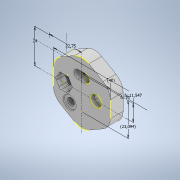
# Autodesk Inventor part: Bottom
Saved by Autodesk Inventor 2022 (Build 260153000, 153)
## iProperties
Created: 2021-02-26
Part Number: Bottom
Material: Generic
Document SubType Name: Modeling
Designer: Viktor
Density: 1 g/cm^3
Appearance: Default
Author: Viktor
Autodesk Inventor part; units mm, degrees
ref_plane "YZ Plane" through (0, 0, 0) normal (1, 0, 0) x (0, 1, 0)
ref_plane "XZ Plane" through (0, 0, 0) normal (0, 1, 0) x (-1, 0, 0)
ref_plane "XY Plane" through (0, 0, 0) normal (0, 0, 1) x (1, 0, 0)
sketch "Sketch1" plane through (0, 0, 0) normal (0, 0, 1) x (1, 0, 0)
  circle A0 centre (0, 0) radius 7.5
  line L0 (-5.7735, 0) -> (-2.8868, 5)
  line L1 (-2.8868, 5) -> (2.8868, 5)
  line L2 (2.8868, 5) -> (5.7735, 0)
  line L3 (5.7735, 0) -> (2.8868, -5)
  line L4 (2.8868, -5) -> (-2.8868, -5)
  line L5 (-2.8868, -5) -> (-5.7735, 0)
  dimension "d0" = 15
  dimension "d1" = 10
  constraints: 12 end point, 2 coincident, 1 centre point, 13 other
  measures "d0" diameter of A0
  measures "d1" distance between parallel lines of L3 L0
extrude "Extrusion1" add sketch "Sketch1" along normal blind 9 contours A0 | L0 L1 L2 L3 L4 L5
sketch "Sketch4" plane through (0, 0, 9) normal (0, 0, 1) x (1, 0, 0)
  circle A0 centre (0, 0) radius 3
  dimension "d15" = 6
  constraints: 1 centre point, 1 coincident
  measures "d15" diameter of A0
extrude "Extrusion4" cut sketch "Sketch4" against normal through all
sketch "Sketch5" plane through (0, 0, 9) normal (0, 0, 1) x (1, 0, 0)
  line L0 (-2.9156, -5.05) -> (-5.8312, 0)
  line L1 (-5.8312, 0) -> (-2.9156, 5.05)
  line L2 (-2.9156, 5.05) -> (2.9156, 5.05)
  line L3 (2.9156, 5.05) -> (5.8312, 0)
  line L4 (5.8312, 0) -> (2.9156, -5.05)
  line L5 (2.9156, -5.05) -> (-2.9156, -5.05)
  point P0 (0, 0)
  point P1 (0, 0)
  dimension "d18" = 10.1
  constraints: 12 end point, 1 coincident, 1 horizontal, 13 other
  measures "d18" distance between parallel lines of L5 L2
extrude "Extrusion5" cut sketch "Sketch5" against normal blind 6
sketch "Sketch6" plane through (0, 0, 9) normal (0, 0, 1) x (1, 0, 0)
  point P0 (0, 0)
fillet "Fillet1" radius 2.1 6 edges at (5.8312, 0, 6) (2.9156, 5.05, 6) (-2.9156, 5.05, 6) (-5.8312, 0, 6) (-2.9156, -5.05, 6) (2.9156, -5.05, 6)
sketch "Sketch7" plane through (0, 0, 9) normal (0, 0, 1) x (1, 0, 0)
  arc A0 (-3.5218, -4) -> (-1.7032, -5.05) centre (-1.7032, -2.95) ccw projected
  arc A1 (-5.225, 1.05) -> (-5.225, -1.05) centre (-3.4064, 0) ccw projected
  arc A2 (-1.7032, 5.05) -> (-3.5218, 4) centre (-1.7032, 2.95) ccw projected
  arc A3 (3.5218, 4) -> (1.7032, 5.05) centre (1.7032, 2.95) ccw projected
  arc A4 (5.225, -1.05) -> (5.225, 1.05) centre (3.4064, 0) ccw projected
  arc A5 (1.7032, -5.05) -> (3.5218, -4) centre (1.7032, -2.95) ccw projected
  line L0 (-45.8, 0) -> (57.8, 0) projected
  circle A6 centre (-4.6441, 0) radius 1.2
  point P0 (0, 0)
  dimension "d22" = 2.4
  constraints: 1 point on line, 3 other
extrude "Extrusion6" cut sketch "Sketch7" against normal up to surface (6 mm away)
pattern_circular "Circular Pattern1" count 6 over 360 about axis through (0, 0, 9) along (0, 0, -1) of "Extrusion6"
sketch "Sketch9" plane through (0, 0, 0) normal (0, 0, 1) x (1, 0, 0)
  line L0 (-10.5, 0) -> (10.5, 0) projected
  circle A0 centre (12.5, 0) radius 20 construction
  circle A1 centre (0, 0) radius 7.5 projected
  line L1 (-7.5, -11.547) -> (-7.5, 11.547)
  line L2 (-7.5, 11.547) -> (12.5, 23.094)
  line L3 (12.5, 23.094) -> (32.5, 11.547)
  line L4 (32.5, 11.547) -> (32.5, -11.547)
  line L5 (32.5, -11.547) -> (12.5, -23.094)
  line L6 (12.5, -23.094) -> (-7.5, -11.547)
  point P0 (-7.5, 0)
  point P1 (-7.5, 0)
  dimension "d28" = 40
  constraints: 12 end point, 2 tangent, 1 centre point, 1 coincident, 1 point on line, 1 vertical, 13 other
  measures "d28" diameter of A0
extrude "Extrusion7" add sketch "Sketch9" along normal up to surface (9 mm away)
sketch "Sketch10" plane through (10, 0, 9) normal (0, 0, 1) x (1, 0, 0)
  circle A0 centre (-6, -10) radius 2 construction
  point P0 (-10, 0)
  dimension "d31" = 4
  dimension "d32" = 4
  dimension "d33" = 10
  constraints: 1 centre point
  measures "d31" diameter of A0
  measures "d32" horizontal distance of point (-10, 0) A0.centre
  measures "d33" vertical distance of point (-10, 0) A0.centre
fillet "Fillet2" radius 10 6 edges at (-7.5, -11.547, 4.5) (12.5, -23.094, 4.5) (32.5, -11.547, 4.5) (-7.5, 11.547, 4.5) (12.5, 23.094, 4.5) (32.5, 11.547, 4.5)
hole "Hole1" at (4, -10, 9) direction (0, 0, -1) diameter 5 end through all counterbore diameter 9 counterbore depth 0.8
sketch "Sketch13" plane through (0, 0, 0) normal (0, 0, -1) x (-1, 0, 0)
  circle A0 centre (-4, -10) radius 2.5 projected
  line L0 (-8.05, -7.6617) -> (-4, -5.3235)
  line L1 (-4, -5.3235) -> (0.05, -7.6617)
  line L2 (0.05, -7.6617) -> (0.05, -12.3383)
  line L3 (0.05, -12.3383) -> (-4, -14.6765)
  line L4 (-4, -14.6765) -> (-8.05, -12.3383)
  line L5 (-8.05, -12.3383) -> (-8.05, -7.6617)
  line L6 (2.5, -14.4338) -> (-7.5, -20.2073) projected
  point P0 (0, 0)
  point P1 (-6.025, -13.5074)
  dimension "d44" = 8.1
  constraints: 12 end point, 1 coincident, 1 midpoint, 1 parallel, 13 other
  measures "d44" distance between parallel lines of L5 L2
extrude "Extrusion9" cut sketch "Sketch13" against normal blind 5.2
fillet "Fillet3" radius 2.1 6 edges at (4, -14.6765, 2.6) (-0.05, -12.3383, 2.6) (-0.05, -7.6617, 2.6) (4, -5.3235, 2.6) (8.05, -7.6617, 2.6) (8.05, -12.3383, 2.6)
sketch "Sketch15" plane through (0, 0, 0) normal (0, 0, -1) x (-1, 0, 0)
  arc A0 (-5.05, -14.0703) -> (-2.95, -14.0703) centre (-4, -12.2517) ccw projected
  line L0 (-4, -12.2517) -> (-4, -11.6129) construction
  circle A1 centre (-4, -13.3921) radius 1.25
  point P0 (0, 0)
  dimension "d48" = 2.5
  constraints: 2 end point, 1 point on line, 1 vertical, 3 other
extrude "Extrusion10" cut sketch "Sketch15" against normal up to surface (5.2 mm away)
pattern_circular "Circular Pattern2" count 6 over 360 about axis through (4, -10, -50.4819) along (0, 0, 1) of "Extrusion10"
sketch "Sketch16" plane through (0, 0, 9) normal (0, 0, 1) x (1, 0, 0)
  circle A0 centre (22.5, 0) radius 4
  line L0 (32.5, 5.7735) -> (32.5, -5.7735) projected
  point P0 (0, 0)
  dimension "d54" = 8
  dimension "d68" = 10
  constraints: 1 centre point
  measures "d54" diameter of A0
  measures "d68" distance from line of L0 A0.centre
extrude "Extrusion11" cut sketch "Sketch16" against normal through all
sketch "Sketch17" plane through (0, 0, 0) normal (0, 0, -1) x (-1, 0, 0)
  circle A0 centre (-22.5, 0) radius 4 projected
  line L0 (-29.05, -3.7816) -> (-29.05, 3.7816)
  line L1 (-29.05, 3.7816) -> (-22.5, 7.5633)
  line L2 (-22.5, 7.5633) -> (-15.95, 3.7816)
  line L3 (-15.95, 3.7816) -> (-15.95, -3.7816)
  line L4 (-15.95, -3.7816) -> (-22.5, -7.5633)
  line L5 (-22.5, -7.5633) -> (-29.05, -3.7816)
  line L6 (-32.5, -5.7735) -> (-32.5, 5.7735) projected
  point P0 (0, 0)
  dimension "d58" = 13.1
  constraints: 12 end point, 1 coincident, 1 parallel, 13 other
  measures "d58" distance between parallel lines of L0 L3
extrude "Extrusion12" cut sketch "Sketch17" against normal blind 5.5
fillet "Fillet4" radius 2.1 6 edges at (22.5, -7.5633, 2.75) (15.95, -3.7816, 2.75) (15.95, 3.7816, 2.75) (22.5, 7.5633, 2.75) (29.05, 3.7816, 2.75) (29.05, -3.7816, 2.75)
sketch "Sketch19" plane through (0, 0, 0) normal (0, 0, -1) x (-1, 0, 0)
  arc A0 (-23.55, -6.9571) -> (-21.45, -6.9571) centre (-22.5, -5.1384) ccw projected
  line L0 (-22.5, -5.1384) -> (-22.5, -8.2461) construction
  circle A1 centre (-22.5, -6.3761) radius 1.2
  arc A2 (-23.55, -6.9571) -> (-21.45, -6.9571) centre (-22.5, -5.1384) ccw projected
  line L1 (-21.45, -6.9571) -> (-22.5, -7.5633) construction
  line L2 (-23.55, -6.9571) -> (-22.5, -7.5633) construction
  line L3 (-23.55, -6.9571) -> (-28, -4.3879) projected
  point P0 (0, 0)
  dimension "d62" = 2.4
  constraints: 6 end point, 3 point on circle, 2 point on line, 2 tangent, 1 centre point, 1 collinear, 1 vertical
  measures "d62" diameter of A1
extrude "Extrusion13" cut sketch "Sketch19" against normal up to surface (5.5 mm away)
pattern_circular "Circular Pattern3" count 6 over 360 about axis through (22.5, 0, 9) along (0, 0, -1) of "Extrusion13"
sketch "Sketch20" plane through (0, 0, 5.5) normal (0, 0, -1) x (-1, 0, 0)
  circle A0 centre (-22.5, 0) radius 4 projected
  circle A1 centre (-22.5, 0) radius 5.9
  point P0 (0, 0)
  dimension "d69" = 11.8
  constraints: 1 centre point, 1 coincident
  measures "d69" diameter of A1
extrude "Extrusion14" cut sketch "Sketch20" against normal blind 0.65
sketch "Sketch21" plane through (0, 0, 9) normal (0, 0, 1) x (1, 0, 0)
  point P0 (0, 0)
sketch "Sketch22" plane through (0, 0, 9) normal (0, 0, 1) x (1, 0, 0)
  line L0 (54.5318, 10) -> (-19.1234, 10) construction
  arc A0 (32.5, 5.7735) -> (27.5, 14.4338) centre (22.5, 5.7735) ccw projected
  line L1 (-7.5, -5.7735) -> (-7.5, 5.7735) projected
  line L2 (15, 10) -> (10, 10) construction
  line L3 (15, 13) -> (10, 13)
  line L4 (10, 7) -> (15, 7)
  arc A1 (15, 7) -> (15, 13) centre (15, 10) ccw
  arc A2 (10, 13) -> (10, 7) centre (10, 10) ccw
  line L5 (12.5, 32) -> (12.5, -41) construction
  point P0 (0, 0)
  point P1 (12.5, 10)
  dimension "d72" = 40
  dimension "d74" = 6
  dimension "d75" = 5
  dimension "d76" = 10
  dimension "d79" = 20
  constraints: 12 end point, 4 point on circle, 4 tangent, 3 point on line, 2 centre point, 1 horizontal, 1 midpoint, 1 parallel, 1 vertical
  measures "d74" distance between parallel lines of L3 L4
  measures "d75" distance of L4.start L4.end
  measures "d76" vertical distance of point (0, 0) point (12.5, 10)
  measures "d79" distance between parallel lines of L1 L5
extrude "Extrusion15" cut sketch "Sketch22" against normal blind 10
sketch "Sketch23" plane through (0, 0, 9) normal (0, 0, 1) x (1, 0, 0)
  arc A0 (15, 7) -> (15, 13) centre (15, 10) ccw projected
  circle A1 centre (22.5, 0) radius 4 projected
  point P0 (0, 0)
sketch "Sketch24" plane through (0, 0, 0) normal (0, 0, -1) x (-1, 0, 0)
  arc A0 (7.5, 5.7735) -> (2.5, 14.4338) centre (-2.5, 5.7735) ccw projected
  line L0 (7.5, 5.7735) -> (7.5, 22) construction
  line L1 (-10, 7) -> (31, 7) construction
  point P0 (0, 0)
  point P1 (7.5, 7)
  constraints: 4 end point, 2 point on line, 1 coincident, 1 horizontal, 1 tangent, 1 vertical
sketch "Sketch25" plane through (0, 0, 9) normal (0, 0, 1) x (1, 0, 0)
  arc A0 (-2.5, 14.4338) -> (-7.5, 5.7735) centre (2.5, 5.7735) ccw projected
  point P0 (0, 0)
  point P1 (-7.5, 7)
sketch "Sketch26" plane through (0, 0, 0) normal (0, 0, -1) x (-1, 0, 0)
  circle A0 centre (-4, -10) radius 2.5 projected
  circle A1 centre (-22.5, 0) radius 4 projected
  circle A2 centre (0, 0) radius 3 projected
sketch "Sketch27" plane through (0, 0, 0) normal (0, 0, -1) x (-1, 0, 0)
  line L0 (-17, -4.3879) -> (-21.45, -6.9571) projected
  arc A0 (-23.55, -6.9571) -> (-21.45, -6.9571) centre (-22.5, -6.3761) ccw projected
  line L1 (-23.55, -6.9571) -> (-28, -4.3879) projected
  arc A1 (-29.05, -2.5692) -> (-28, -4.3879) centre (-28.0219, -3.1881) ccw projected
  line L2 (-29.05, -2.5692) -> (-29.05, 2.5692) projected
  arc A2 (-28, 4.3879) -> (-29.05, 2.5692) centre (-28.0219, 3.1881) ccw projected
  line L3 (-28, 4.3879) -> (-23.55, 6.9571) projected
  arc A3 (-21.45, 6.9571) -> (-23.55, 6.9571) centre (-22.5, 6.3761) ccw projected
  line L4 (-21.45, 6.9571) -> (-17, 4.3879) projected
  arc A4 (-15.95, 2.5692) -> (-17, 4.3879) centre (-16.9781, 3.1881) ccw projected
  line L5 (-15.95, 2.5692) -> (-15.95, -2.5692) projected
  arc A5 (-17, -4.3879) -> (-15.95, -2.5692) centre (-16.9781, -3.1881) ccw projected
  line L6 (-1, -12.9445) -> (-2.95, -14.0703) projected
  arc A6 (-5.05, -14.0703) -> (-2.95, -14.0703) centre (-4, -13.3921) ccw projected
  line L7 (-5.05, -14.0703) -> (-7, -12.9445) projected
  arc A7 (-8.05, -11.1258) -> (-7, -12.9445) centre (-6.9376, -11.696) ccw projected
  line L8 (-8.05, -11.1258) -> (-8.05, -8.8742) projected
  arc A8 (-7, -7.0555) -> (-8.05, -8.8742) centre (-6.9376, -8.304) ccw projected
  line L9 (-7, -7.0555) -> (-5.05, -5.9297) projected
  arc A9 (-2.95, -5.9297) -> (-5.05, -5.9297) centre (-4, -6.6079) ccw projected
  line L10 (-2.95, -5.9297) -> (-1, -7.0555) projected
  arc A10 (0.05, -8.8742) -> (-1, -7.0555) centre (-1.0624, -8.304) ccw projected
  line L11 (0.05, -8.8742) -> (0.05, -11.1258) projected
  arc A11 (-1, -12.9445) -> (0.05, -11.1258) centre (-1.0624, -11.696) ccw projected
  point P0 (0, 0)
sketch "Sketch28" plane through (0, 0, 9) normal (0, 0, 1) x (1, 0, 0)
  line L0 (-16.3382, 0) -> (43, 0) construction
  line L1 (12.5, 25) -> (12.5, -25) construction
  line L2 (32.5, 5.7735) -> (32.5, -5.7735) projected
  line L3 (-7.5, -5.7735) -> (-7.5, 5.7735) projected
  arc A0 (7.5, -20.2073) -> (17.5, -20.2073) centre (12.5, -11.547) ccw projected
  arc A1 (17.5, 20.2073) -> (7.5, 20.2073) centre (12.5, 11.547) ccw projected
  point P0 (0, 0)
  point P1 (-10.25, 24)
  dimension "d80" = 40
  dimension "d81" = 20
  dimension "d82" = 23.094
  dimension "d83" = 11.547
  dimension "d84" = 22.75
  dimension "d85" = 24
  constraints: 4 end point, 1 horizontal
  measures "d80" distance between parallel lines of L2 L3
  measures "d81" distance between parallel lines of L2 L1
  measures "d82" distance of A0.centre A1.centre
  measures "d83" distance from line of A1.centre L0
  measures "d84" distance from line of L1 point (-10.25, 24)
  measures "d85" distance from line of L0 point (-10.25, 24)
equation "\"d79\" = 0.5 * d72"
equation "\"d81\" = 0.5 * d80"
equation "\"d83\" = 0.5 * d82"
body "Solid1"
